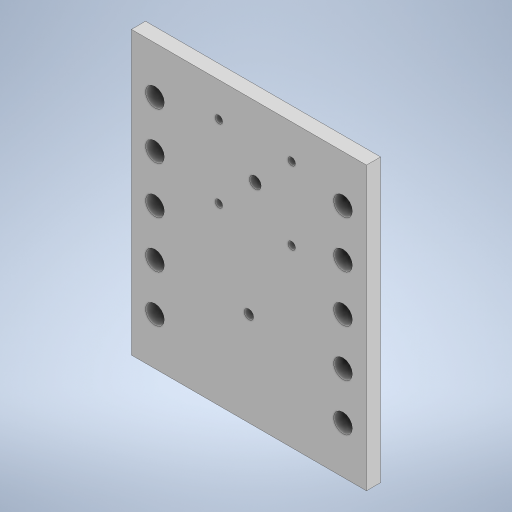
# Autodesk Inventor part: motor_gear_holder
Saved by Autodesk Inventor 2023 (Build 270158000, 158)
## iProperties
Created: 2022-07-08
Part Number: motor_gear_holder
Material: Generic
Document SubType Name: Modeling
Designer: Zayed
Density: 1 g/cm^3
Appearance: Default
Author: Zayed
Autodesk Inventor part; units mm, degrees
ref_plane "YZ Plane" through (0, 0, 0) normal (1, 0, 0) x (0, 1, 0)
ref_plane "XZ Plane" through (0, 0, 0) normal (0, 1, 0) x (-1, 0, 0)
ref_plane "XY Plane" through (0, 0, 0) normal (0, 0, 1) x (1, 0, 0)
ref_plane "Work Plane1" through (0, 0, 0) normal (0, 0, 1) x (1, 0, 0)
sketch "Sketch1" plane through (0, 0, 0) normal (0, 0, 1) x (1, 0, 0)
  circle A0 centre (29.5896, 9.9505) radius 2
  circle A1 centre (32.2876, 59.8777) radius 2.5
  line L0 (29.5896, 9.9505) -> (29.5896, -30.0495)
  line L1 (29.5896, -30.0495) -> (79.5896, -30.0495)
  line L2 (79.5896, -30.0495) -> (79.5896, 89.9505)
  line L3 (79.5896, 89.9505) -> (-20.4104, 89.9505)
  line L4 (-20.4104, 89.9505) -> (79.5896, 89.9505)
  line L5 (79.5896, 89.9505) -> (79.5896, -30.0495)
  line L6 (79.5896, -30.0495) -> (-20.4104, -30.0495)
  line L7 (-20.4104, -30.0495) -> (-20.4104, 89.9505)
  circle A2 centre (16.7876, 75.3777) radius 1.6
  circle A3 centre (47.7876, 75.3777) radius 1.6
  circle A4 centre (47.7876, 44.3777) radius 1.6
  circle A5 centre (16.7876, 44.3777) radius 1.6
  line L8 (-20.4104, 89.9505) -> (-10.4104, 89.9505)
  line L9 (-10.4104, 89.9505) -> (-10.4104, 69.9505)
  line L10 (-10.4104, 69.9505) -> (-10.4104, 49.9505)
  line L11 (-10.4104, 49.9505) -> (-10.4104, 29.9505)
  line L12 (-10.4104, 29.9505) -> (-10.4104, 9.9505)
  line L13 (-10.4104, 9.9505) -> (-10.4104, -10.0495)
  line L14 (79.5896, 89.9505) -> (69.5896, 89.9505)
  line L15 (69.5896, 89.9505) -> (69.5896, 69.9505)
  line L16 (69.5896, 69.9505) -> (69.5896, 49.9505)
  line L17 (69.5896, 49.9505) -> (69.5896, 29.9505)
  line L18 (69.5896, 29.9505) -> (69.5896, 9.9505)
  line L19 (69.5896, 9.9505) -> (69.5896, -10.0495)
  circle A6 centre (-10.4104, 69.9505) radius 4
  circle A7 centre (-10.4104, 49.9505) radius 4
  circle A8 centre (-10.4104, 29.9505) radius 4
  circle A9 centre (-10.4104, 9.9505) radius 4
  circle A10 centre (-10.4104, -10.0495) radius 4
  circle A11 centre (69.5896, 69.9505) radius 4
  circle A12 centre (69.5896, 49.9505) radius 4
  circle A13 centre (69.5896, 29.9505) radius 4
  circle A14 centre (69.5896, 9.9505) radius 4
  circle A15 centre (69.5896, -10.0495) radius 4
  dimension "d0" = 4
  dimension "d1" = 5
  dimension "d2" = 40
  dimension "d3" = 50
  dimension "d4" = 120
  dimension "d5" = 100
  dimension "d6" = 3.2
  dimension "d7" = 3.2
  dimension "d8" = 3.2
  dimension "d9" = 3.2
  dimension "d10" = 10
  dimension "d11" = 20
  dimension "d12" = 20
  dimension "d13" = 20
  dimension "d14" = 20
  dimension "d15" = 20
  dimension "d16" = 10
  dimension "d17" = 20
  dimension "d18" = 20
  dimension "d19" = 20
  dimension "d20" = 20
  dimension "d21" = 20
  dimension "d22" = 8
  dimension "d23" = 8
  dimension "d24" = 8
  dimension "d25" = 8
  dimension "d26" = 8
  dimension "d27" = 8
  dimension "d28" = 8
  dimension "d29" = 8
  dimension "d30" = 8
  dimension "d31" = 8
  constraints: 40 end point, 16 centre point, 10 coincident, 9 point on line, 6 perpendicular, 2 parallel, 2 vertical, 1 horizontal
  measures "d0" diameter of A0
  measures "d1" diameter of A1
  measures "d2" distance of L0.start L0.end
  measures "d3" distance of L0.end L1.end
  measures "d4" distance of L1.end L2.end
  measures "d5" distance of L2.end L3.end
  measures "d6" diameter of A2
  measures "d7" diameter of A3
  measures "d8" diameter of A4
  measures "d9" diameter of A5
  measures "d10" distance of L3.end L8.end
  measures "d11" distance of L8.end L9.end
  measures "d12" distance of L9.end L10.end
  measures "d13" distance of L10.end L11.end
  measures "d14" distance of L11.end L12.end
  measures "d15" distance of L12.end L13.end
  measures "d16" distance of L4.end L14.end
  measures "d17" distance of L14.end L15.end
  measures "d18" distance of L15.end L16.end
  measures "d19" distance of L16.end L17.end
  measures "d20" distance of L17.end L18.end
  measures "d21" distance of L18.end L19.end
  measures "d22" diameter of A6
  measures "d23" diameter of A7
  measures "d24" diameter of A8
  measures "d25" diameter of A9
  measures "d26" diameter of A10
  measures "d27" diameter of A11
  measures "d28" diameter of A12
  measures "d29" diameter of A13
  measures "d30" diameter of A14
  measures "d31" diameter of A15
extrude "Extrusion1" add sketch "Sketch1" along normal blind 6
body "Solid1"
